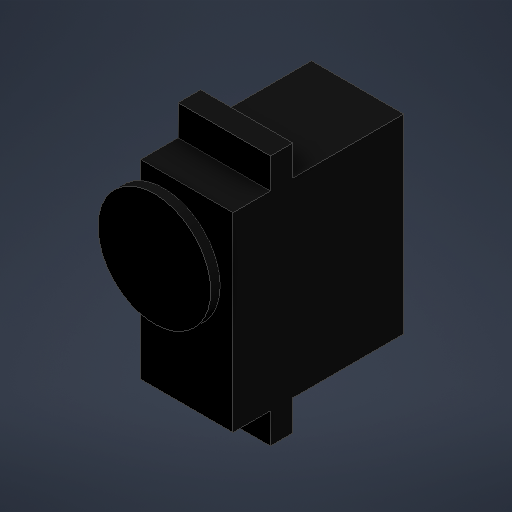
# Autodesk Inventor part: Servo
Saved by Autodesk Inventor 2025 (Build 290162000, 162)
## iProperties
Created: 2024-04-22
Part Number: Servo
Material: Generic
Document SubType Name: Modeling
Designer: conno
Density: 1 g/cm^3
Appearance: Default
ServoWidth: 0.770 in
ServoHeight: 1.588 in
ServoLength: 1.426 in
ServoTabWidth: 0.188 in
ServoTabHeight: 0.254 in
ServoTabDepthOffset: 0.313 in
ServoWheelDiameter: 0.941 in
Author: conno
Autodesk Inventor part; units mm, degrees
ref_plane "YZ Plane" through (0, 0, 0) normal (1, 0, 0) x (0, 1, 0)
ref_plane "XZ Plane" through (0, 0, 0) normal (0, 1, 0) x (-1, 0, 0)
ref_plane "XY Plane" through (0, 0, 0) normal (0, 0, 1) x (1, 0, 0)
sketch "Sketch1" plane through (0, 0, 0) normal (0, 0, 1) x (1, 0, 0)
  line L0 (-9.779, -20.1676) -> (9.779, -20.1676)
  line L1 (9.779, -20.1676) -> (9.779, 20.1676)
  line L2 (9.779, 20.1676) -> (-9.779, 20.1676)
  line L3 (-9.779, 20.1676) -> (-9.779, -20.1676)
  line L4 (-9.779, -20.1676) -> (9.779, 20.1676) construction
  line L5 (9.779, -20.1676) -> (-9.779, 20.1676) construction
  point P0 (0, 0)
  dimension "ServoWidth" = 19.558
  dimension "ServoHeight" = 40.3352
  constraints: 12 end point, 2 midpoint, 2 parallel, 1 horizontal, 1 perpendicular
  measures "ServoWidth" distance of L2.end L1.end
  measures "ServoHeight" distance of L1.end L0.end
extrude "Body" add sketch "Sketch1" along normal mid plane 36.2077
sketch "Sketch2" plane through (0, 0, 18.1038) normal (0, 0, 1) x (1, 0, 0)
  circle A0 centre (0, 10.2616) radius 4.4259
  line L0 (9.779, 20.1676) -> (-9.779, 20.1676) projected
  point P0 (0, 0)
  dimension "d4" = 8.8519
  dimension "d7" = 9.906
  constraints: 1 centre point, 1 vertical alignment
  measures "d4" diameter of A0
  measures "d7" distance from line of L0 A0.centre
extrude "Actuator" add sketch "Sketch2" along normal blind 4.8514
sketch "Sketch3" plane through (0, 10.2616, 22.9552) normal (0, 0, 1) x (1, 0, 0)
  circle A0 centre (0, 0) radius 11.9444
  point P0 (0, -10.2616)
  dimension "ServoWheelDiameter" = 23.8887
  constraints: 1 centre point
  measures "ServoWheelDiameter" diameter of A0
extrude "Wheel" add sketch "Sketch3" along normal blind 2.0193
sketch "Sketch4" plane through (-9.779, -20.1676, 18.1038) normal (-1, 0, 0) x (0, 0, 1)
  line L0 (-7.9375, -6.4389) -> (-12.7, -6.4389)
  line L1 (-12.7, -6.4389) -> (-12.7, 0)
  line L2 (-12.7, 0) -> (-7.9375, 0)
  line L3 (-7.9375, 0) -> (-7.9375, -6.4389)
  line L4 (-7.9375, -6.4389) -> (-12.7, 0) construction
  line L5 (-12.7, -6.4389) -> (-7.9375, 0) construction
  line L6 (-36.2077, 0) -> (0, 0) projected
  line L7 (0, 40.3352) -> (0, 0) projected
  line L8 (-12.7, 46.7741) -> (-7.9375, 46.7741)
  line L9 (-7.9375, 46.7741) -> (-7.9375, 40.3352)
  line L10 (-7.9375, 40.3352) -> (-12.7, 40.3352)
  line L11 (-12.7, 40.3352) -> (-12.7, 46.7741)
  line L12 (-12.7, 46.7741) -> (-7.9375, 40.3352) construction
  line L13 (-7.9375, 46.7741) -> (-12.7, 40.3352) construction
  line L14 (-36.2077, 40.3352) -> (0, 40.3352) projected
  point P0 (-18.1038, 20.1676)
  point P1 (-10.3188, -3.2195)
  point P2 (-10.3188, 43.5546)
  point P3 (-7.9375, 43.5546)
  point P4 (-7.9375, -3.2194)
  dimension "ServoTabWidth" = 4.7625
  dimension "ServoTabHeight" = 6.4389
  dimension "ServoTabDepthOffset" = 7.9375
  dimension "d16" = 6.4389
  dimension "d17" = 4.7625
  constraints: 24 end point, 6 midpoint, 4 parallel, 2 collinear, 2 horizontal, 2 perpendicular, 1 vertical alignment
  measures "ServoTabWidth" distance of L1.end L2.end
  measures "ServoTabHeight" distance of L0.end L1.end
  measures "ServoTabDepthOffset" distance between parallel lines of L7 L3
  measures "d16" distance of L8.end L9.end
  measures "d17" distance of L9.end L10.end
extrude "Tabs" add sketch "Sketch4" against normal up to surface (19.558 mm away)
equation "\"d16\" = ServoTabHeight"
equation "\"d17\" = ServoTabWidth"
body "Solid1"
